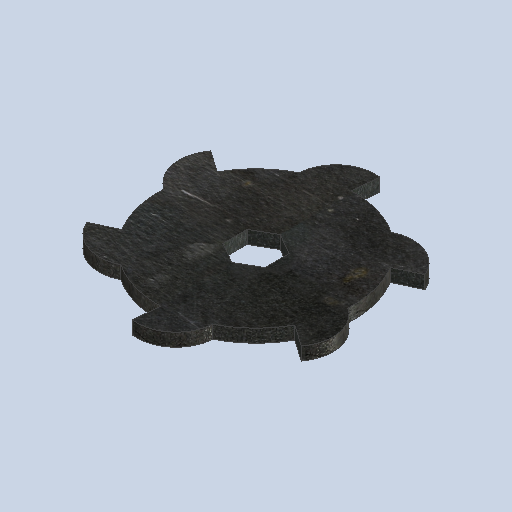
# Autodesk Inventor part: NVPH-203 shredder cutter blade 3
Saved by Autodesk Inventor 2025 (Build 290162010, 162A)
## iProperties
Created: 2024-12-04
Part Number: NVPH-203 shredder cutter blade 3
Material: Steel
Document SubType Name: Sheet Metal
Designer: DELL
Density: 7.85 g/cm^3
Appearance: Plate
Sheet Metal Rule: Default_mm
Mass: 1581.58 g
Surface Area: 482.858 cm^2
Volume: 201.476 cm^3
Flat Pattern Width: 18.1485 cm
Flat Pattern Length: 18.9326 cm
Flat Pattern Area: 343.598 cm^2
Sheet Metal Width: 181,485 mm
Sheet Metal Length: 189,326 mm
Sheet Metal Area: 34359,831 mm^2
Author: DELL
Autodesk Inventor part; units mm, degrees
ref_plane "YZ Plane" through (0, 0, 0) normal (1, 0, 0) x (0, 1, 0)
ref_plane "XZ Plane" through (0, 0, 0) normal (0, 1, 0) x (-1, 0, 0)
ref_plane "XY Plane" through (0, 0, 0) normal (0, 0, 1) x (1, 0, 0)
sketch "Sketch1" plane through (0, 0, 0) normal (0, 0, 1) x (1, 0, 0)
  line L0 (0, -18.5907) -> (-16.1, -9.2953)
  line L1 (-16.1, -9.2953) -> (-16.1, 9.2953)
  line L2 (-16.1, 9.2953) -> (0, 18.5907)
  line L3 (0, 18.5907) -> (16.1, 9.2953)
  line L4 (16.1, 9.2953) -> (16.1, -9.2953)
  line L5 (16.1, -9.2953) -> (0, -18.5907)
  circle A0 centre (0, 0) radius 100
  circle A1 centre (0, 0) radius 75
  line L6 (0, 0) -> (-55.1345, 0)
  dimension "d0" = 32.2
  dimension "d1" = 200
  dimension "d2" = 150
  dimension "d14" = 30
  constraints: 14 end point, 3 coincident, 2 centre point, 1 horizontal, 13 other
  measures "d0" distance between parallel lines of L5 L2
  measures "d1" diameter of A0
  measures "d2" diameter of A1
  measures "d14" angle of L6 L5
extrude "Extrusion1" add sketch "Sketch1" along normal blind 10 contours A1
sketch "Sketch2" plane through (0, 0, 0) normal (0, 0, 1) x (1, 0, 0)
  circle A0 centre (0, 0) radius 75 projected
  line L0 (0, 0) -> (0, 75) construction
  line L1 (0, 95) -> (-15.0761, 73.4691) construction
  line L2 (0, 95) -> (-1.7516, 74.9795)
  circle A1 centre (0, 0) radius 75 projected
  arc A2 (0, 95) -> (-33.7647, 66.9697) centre (-3.8144, 65.2435) ccw
  line L3 (0, 75) -> (0, 95) construction
  point P0 (-1.7516, 74.9795)
  point P1 (-33.7647, 66.9697)
  dimension "d5" = 5
  dimension "d8" = 35
  dimension "d15" = 30
  dimension "d16" = 33
  dimension "d17" = 20
  constraints: 8 end point, 5 point on circle, 2 vertical, 1 centre point, 2 other
  measures "d5" angle of L2 L0
  measures "d8" angle of L0 L1
  measures "d15" radius of A2
  measures "d16" distance of A2.end L2.end
  measures "d17" distance of L0.end L1.start
extrude "Extrusion2" add sketch "Sketch2" along normal blind 10 contours A0 A2 L2
pattern_circular "Circular Pattern1" count 6 over 360 about axis through (0, 0, -10) along (0, 0, 1) of "Extrusion2"
equation "\"BendReliefDepth\" = 0.5 * Thickness"
equation "\"Thickness\" = 10"
body "Solid1"
